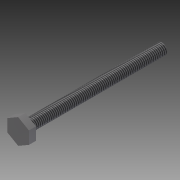
# Autodesk Inventor part: Fi3es60mmcsavar
Saved by Autodesk Inventor 2015 SP1 (Build 190203100, 203)
## iProperties
Created: 2014-11-03
Part Number: Fi3es60mmcsavar
Material: Steel, Alloy
Document SubType Name: Modeling
Designer: laca
Density: 7.73 g/cm^3
Appearance: Semi-Polished
Mass: 2.55832 g
Surface Area: 4.62065 cm^2
Volume: 0.33096 cm^3
Author: laca
Autodesk Inventor part; units mm, degrees
ref_plane "YZ Plane" through (0, 0, 0) normal (1, 0, 0) x (0, 1, 0)
ref_plane "XZ Plane" through (0, 0, 0) normal (0, 1, 0) x (-1, 0, 0)
ref_plane "XY Plane" through (0, 0, 0) normal (0, 0, 1) x (1, 0, 0)
sketch "Sketch1" plane through (0, 0, 0) normal (0, 1, 0) x (-1, 0, 0)
  line L0 (0, 3.9544) -> (10, 3.9544)
  line L1 (1.5, 1.9544) -> (1.5, -36.0456)
  line L2 (1.5, -36.0456) -> (0, -36.0456)
  line L3 (0, -36.0456) -> (0, 3.9544)
  line L4 (1.5, 1.9544) -> (10, 1.9544)
  line L5 (10, 3.9544) -> (10, 1.9544)
  point P0 (0, 0)
  dimension "d0" = 10
  dimension "d1" = 2
  dimension "d2" = 40
  dimension "d21" = 1.5
  constraints: 12 end point, 4 perpendicular, 2 horizontal
  measures "d0" distance of L0.start L0.end
  measures "d1" distance from line of L1.start L0
  measures "d2" distance between parallel lines of L2 L0
  measures "d21" distance between parallel lines of L3 L1
revolve "Revolution1" add sketch "Sketch1" angle 360 about axis through (0, 0, -36.0456) along (0, 0, 1)
thread "Thread2" size "M3x0.5" class "6g" standard "ANSI Metric M Profile" full length
sketch "Sketch5" plane through (0, 0, 3.9544) normal (0, 0, 1) x (1, 0, 0)
  line L0 (-3.0066, 1.7206) -> (-0.0132, 3.4641)
  line L1 (-0.0132, 3.4641) -> (2.9934, 1.7435)
  line L2 (2.9934, 1.7435) -> (3.0066, -1.7206)
  line L3 (3.0066, -1.7206) -> (0.0132, -3.4641)
  line L4 (0.0132, -3.4641) -> (-2.9934, -1.7435)
  line L5 (-2.9934, -1.7435) -> (-3.0066, 1.7206)
  circle A0 centre (0, 0) radius 18.6664
  dimension "d24" = 6
  constraints: 12 end point, 2 coincident, 1 centre point, 13 other
  measures "d24" distance between parallel lines of L2 L5
extrude "Extrusion1" cut sketch "Sketch5" against normal through all
body "Solid1"
